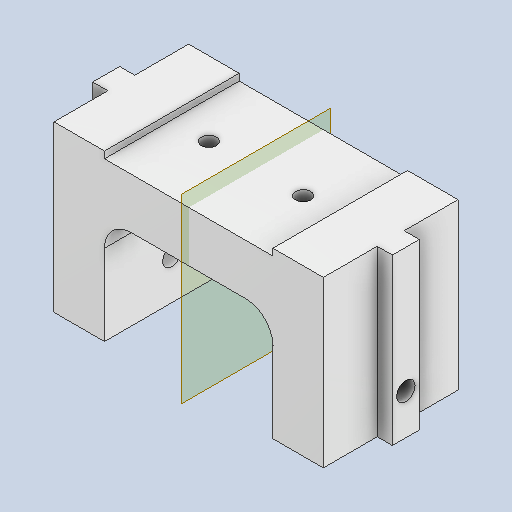
# Autodesk Inventor part: Motor_MainAxis_Frame_Fixation
Saved by Autodesk Inventor 2022 (Build 260153000, 153)
## iProperties
Created: 2022-08-01
Part Number: Motor_MainAxis_Frame_Fixation
Material: PBT-Kunststoff
Document SubType Name: Modeling
Designer: alexw
Density: 1.31 g/cm^3
Appearance: Glatt - Weiß
Mass: 120.55 g
Surface Area: 192.256 cm^2
Volume: 92.0231 cm^3
Author: alexw
Autodesk Inventor part; units mm, degrees
ref_plane "YZ Plane" through (0, 0, 0) normal (1, 0, 0) x (0, 1, 0)
ref_plane "XZ Plane" through (0, 0, 0) normal (0, 1, 0) x (-1, 0, 0)
ref_plane "XY Plane" through (0, 0, 0) normal (0, 0, 1) x (1, 0, 0)
sketch "Skizze1" plane through (0, 0, 0) normal (0, 0, 1) x (1, 0, 0)
  line L0 (25, 49) -> (40, 49)
  line L1 (40, 49) -> (40, 0)
  line L2 (40, 0) -> (25, 0)
  line L3 (25, 0) -> (25, 24)
  line L4 (17, 32) -> (0, 32)
  line L5 (0, 32) -> (0, 0) construction
  line L6 (0, -9.8) -> (0, 58.8) construction
  line L7 (-56, 0) -> (56, 0) construction
  line L8 (0, 47) -> (25, 47)
  line L9 (25, 47) -> (25, 49)
  arc A0 (25, 24) -> (17, 32) centre (17, 24) ccw
  line L10 (25, 12) -> (40, 12) construction
  line L11 (-25, 49) -> (-40, 49)
  line L12 (-40, 49) -> (-40, 0)
  line L13 (-40, 0) -> (-25, 0)
  line L14 (-25, 0) -> (-25, 24)
  line L15 (-17, 32) -> (0, 32)
  line L16 (0, 47) -> (-25, 47)
  line L17 (-25, 47) -> (-25, 49)
  arc A1 (-17, 32) -> (-25, 24) centre (-17, 24) ccw
  line L18 (-25, 12) -> (-40, 12) construction
  line L19 (25, 14.5) -> (40, 14.5) construction
  line L20 (40, 14.5) -> (40, 9.5) construction
  line L21 (40, 9.5) -> (25, 9.5) construction
  line L22 (25, 9.5) -> (25, 14.5) construction
  dimension "d0" = 15
  dimension "d1" = 2
  dimension "d2" = 80
  dimension "d4" = 50
  dimension "d5" = 8
  dimension "d6" = 12
  dimension "d7" = 15
  dimension "d8" = 5
  constraints: 42 end point, 10 symmetric about line, 9 perpendicular, 4 point on circle, 3 midpoint, 3 point on line, 2 centre point, 2 collinear, 2 horizontal, 2 parallel, 2 tangent, 1 other
  measures "d0" distance between parallel lines of L1 L3
  measures "d1" distance between parallel lines of L0 L8
  measures "d2" diameter of L1 L5
  measures "d4" diameter of L9 L5
  measures "d5" radius of A0
  measures "d6" distance between parallel lines of L10 L7
  measures "d7" distance between parallel lines of L4 L8
  measures "d8" distance between parallel lines of L19 L21
extrude "Extrusion1" add sketch "Skizze1" along normal blind 40
sketch "Skizze2" plane through (-25, 47, 0) normal (0, 1, 0) x (1, 0, 0)
  line L0 (50, 0) -> (0, 0) construction
  line L1 (0, 0) -> (0, -40) construction
  line L2 (50, -40) -> (0, -40) construction
  line L3 (50, 0) -> (50, -40) construction
  line L4 (0, 0) -> (0, -40) construction
  line L5 (0, -20) -> (50, -20) construction
  line L6 (50, 0) -> (50, -40) construction
  line L7 (25, -20) -> (25, -40) construction
  line L8 (50, -40) -> (0, -40) construction
  point P0 (25, 0)
  point P1 (11, -20)
  point P2 (39, -20)
  dimension "d11" = 14
  dimension "d12" = 14
  constraints: 4 end point, 4 midpoint, 2 point on line
  measures "d11" distance from line of L7 point (11, -20)
  measures "d12" distance of point (39, -20) L7.start
hole "Bohrung1" at (-14, 47, 20) at (14, 47, 20) direction (0, -1, 0) diameter 4.5 end through all clearance for "Sechskantkopfschraube DIN EN 24017" size "M4" standard "DIN"
sketch "Skizze3" plane through (-40, 0, 0) normal (-1, 0, 0) x (0, 0, 1)
  line L0 (0, 24) -> (0, 0) construction
  line L1 (0, 0) -> (40, 0) construction
  line L2 (40, 24) -> (40, 0) construction
  line L3 (0, 24) -> (40, 24) construction
  line L4 (0, 24) -> (40, 24) construction
  line L5 (20, 24) -> (20, 12) construction
  line L6 (20, 12) -> (40, 12) construction
  point P0 (0, 0)
  constraints: 4 end point, 2 midpoint, 1 coincident, 1 perpendicular, 1 vertical
hole "Bohrung2" at (-40, 12, 20) direction (1, 0, 0) diameter 5.5 end through all clearance for "Sechskantkopfschraube DIN EN 24017" size "M5" standard "DIN"
sketch "Skizze4" plane through (40, 0, 0) normal (1, 0, 0) x (0, 0, -1)
  circle A0 centre (-20, 12) radius 2.75 construction
  line L0 (0, 0) -> (0, 49) construction
  line L1 (0, 49) -> (-40, 49) construction
  line L2 (-40, 0) -> (-40, 49) construction
  line L3 (0, 0) -> (-40, 0) construction
  line L4 (0, 0) -> (-40, 0) construction
  line L5 (-20, 0) -> (-20, 49) construction
  line L6 (-24, 49) -> (-16, 49)
  line L7 (-16, 49) -> (-16, 0)
  line L8 (-16, 0) -> (-24, 0)
  line L9 (-24, 0) -> (-24, 49)
  line L10 (-24, 49) -> (-16, 0) construction
  line L11 (-16, 49) -> (-24, 0) construction
  point P0 (-20, 24.5)
  dimension "d28" = 8
  constraints: 14 end point, 5 midpoint, 2 parallel, 1 horizontal, 1 perpendicular, 1 point on line
  measures "d28" distance between parallel lines of L7 L9
extrude "Extrusion2" add sketch "Skizze4" along normal blind 4.5
ref_plane "Arbeitsebene1" through (0, 0, 0) normal (-1, 0, 0) x (0, 0, 1)
mirror "Spiegeln1" about plane through (0, 0, 0) normal (-1, 0, 0) of "Extrusion2"
delete faces "Fläche löschen1" heal yes whole lump no faces at (40, 10.7843, 19.0833)
delete faces "Fläche löschen2" heal yes whole lump no faces at (-40, 12.2194, 20.89)
equation "\"d2\" = Motor_Frame_FixationPlate_Width"
equation "\"d4\" = Fixation_Width"
equation "\"d9\" = Fixation_Thickness"
equation "\"d11\" = 0.5 * FixationHole_Dist"
equation "\"d12\" = d11"
equation "\"Motor_Frame_FixationPlate_Width\" = 80"
equation "\"Fixation_Width\" = 50"
equation "\"Fixation_Thickness\" = 40"
equation "\"FixationHole_Dist\" = 28"
